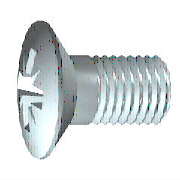
# Autodesk Inventor part: AS 1427 - M6 x 16
Saved by Autodesk Inventor 2016 (Build 200138000, 138)
## iProperties
Created: 2015-02-19
Part Number: AS 1427 - M6 x 16
Material: Steel, Mild
Description: Phillips ISO machine screws
Document SubType Name: Modeling
Standard: AS 1427
Designer: Kenneth Daniel
Standards Organization: AS
Language: en-US
Size Designation: M6 x 16
Categories: <MemberInstance><Categories><Category DisplayName="Fasteners" InternalName="e4da775c-781d-43d5-af7c-5136215cf5a6" Mnemonic="FSTN"><Category DisplayName="Bolts" InternalName="536e6df0-f778-49ac-b2f2-25c71d2aa0b2" Mnemonic="SCRW"><CategoryParameter DisplayName="Nominal Diameter Designation" InternalName="03caf894-eafd-4c09-a035-916ac084b87b" Mnemonic="nomdiadesig"/><CategoryParameter DisplayName="Nominal Length" InternalName="238ecbaf-3e6c-45dd-aa95-4068c8e0fd02" Mnemonic="nomlen"/><CategoryParameter DisplayName="Thread Designation" InternalName="586d5e89-370a-4089-914f-0110033585c7" Mnemonic="thrdesign"/><CategoryParameter DisplayName="Thread Series Designation" InternalName="87c5849c-b3a5-4c3e-9c9b-2feecef9be86" Mnemonic="thrserdsgn"/><CategoryParameter DisplayName="Nominal Diameter" InternalName="8bbe3f8e-44cf-40a9-a251-3a6edc8168d6" Mnemonic="nomdia"/><CategoryParameter DisplayName="Thread Type" InternalName="b4bbb7bc-d6aa-4c9f-a9a9-4152b9f6fe49" Mnemonic="thrtype"/><CategoryParameter DisplayName="Thread Pitch" InternalName="bb82302e-82d8-4176-8fc1-c5d7bb17d5ad" Mnemonic="pitch1"/><CategoryParameter DisplayName="Threads per Unit" InternalName="bdc6e7d2-ffd0-4d9c-a173-16b95ebb912d" Mnemonic="thrperunit1"/><CategoryParameter DisplayName="Thread Class" InternalName="ebc0d23b-2cc6-4d2a-b376-d52aae53bab6" Mnemonic="thrclss"/><Category DisplayName="Countersunk" InternalName="49656530-5684-4604-a233-68d537625f23" Mnemonic="CSSCRW"><CategoryParameter DisplayName="Type" InternalName="161b33bb-bee3-4fab-a17d-97511dff40f0" Mnemonic="type"/><CategoryParameter DisplayName="Thread Length" InternalName="207f0278-6dec-43ab-bffc-1c6d03e64de4" Mnemonic="thrlen"/><CategoryParameter DisplayName="Grip Length" InternalName="2fff3de5-ce2a-45fd-9425-99ddc9dff352" Mnemonic="grplen"/><CategoryParameter DisplayName="Property Class" InternalName="5249b721-5ecc-4781-a2e8-d7e3bda3ecca" Mnemonic="propclss"/><CategoryParameter DisplayName="Head Height" InternalName="57526df9-da71-45fb-acb4-1d0529a34778" Mnemonic="headh"/><CategoryParameter DisplayName="Shank Diameter" InternalName="7ece923f-d8ee-40d5-83f8-980cad520964" Mnemonic="grpdia"/><CategoryParameter DisplayName="Head Diameter" InternalName="a509cd31-06d1-44c5-b54e-d7a695352906" Mnemonic="headdia"/><CategoryParameter DisplayName="Head Angle" InternalName="dbcfc1e0-7990-403e-bc2e-90d1c639222a" Mnemonic="headang"/></Category></Category></Category><Category DisplayName="DataType" InternalName="23b78d0f-2648-40c6-8793-ca6db495c9e8" Mnemonic="DATATYPE"><CategoryParameter DisplayName="DisplayName" InternalName="05415f3d-3907-474b-a020-eb9d644f4cf3" Mnemonic="DISPLAYNAME"/><CategoryParameter DisplayName="Standard" InternalName="0c0a119c-1e12-4c84-803f-101930972f5e" Mnemonic="STANDARD"/><CategoryParameter DisplayName="Description" InternalName="13903e3d-64b1-4950-80da-f627842ea37f" Mnemonic="DESCRIPTION"/><CategoryParameter DisplayName="Designation" InternalName="2675968c-4ce5-49e0-a4f5-552d29089031" Mnemonic="DESIGNATION"/><CategoryParameter DisplayName="Default Row" InternalName="2af9ec52-faaa-4026-b378-f9fa4afca842" Mnemonic="DEFAULTROW"/><CategoryParameter DisplayName="Folder Name" InternalName="3f06958e-8713-4116-9be7-ed6184ecc97b" Mnemonic="FOLDERNAME"/><CategoryParameter DisplayName="Revision Guid" InternalName="45a75005-10b1-4dfc-8d6d-dfe629f0b93c" Mnemonic="REVISIONGUID"/><CategoryParameter DisplayName="FileName" InternalName="8b46a4cc-9585-4fed-90c3-899f57e09a73" Mnemonic="FILENAME"/><CategoryParameter DisplayName="StdsOrg" InternalName="8f5914e1-4693-403f-8ab5-d37768198c9d" Mnemonic="STDSORG"/><CategoryParameter DisplayName="Family Version" InternalName="914462f6-6e19-4b14-ba84-155b9680b1d0" Mnemonic="FAMILYREVISION"/><CategoryParameter DisplayName="Standard Revision" InternalName="91d5a463-65c2-4fde-b823-3b7fea5e8e17" Mnemonic="STANDARDREVISION"/><CategoryParameter DisplayName="Member Revision" InternalName="a65d44b9-392f-4f4f-857b-e4b3d54996fe" Mnemonic="MEMBERREVISION"/><CategoryParameter DisplayName="ClipFormat" InternalName="bc51e27b-3422-4e78-93ef-cec197ddf230" Mnemonic="CLIPFORMAT"/><CategoryParameter DisplayName="Manufacturer" InternalName="cd6c7a72-a28a-4e50-99a9-2c7f4e13e5ad" Mnemonic="MANUFACTURER"/><CategoryParameter DisplayName="InternalName" InternalName="cf1d0246-76d9-4b4a-8305-fa0409afb5c1" Mnemonic="INTERNALNAME"/><CategoryParameter DisplayName="IsMetric" InternalName="e2385c5b-1ea4-4823-96a8-8de651266ec3" Mnemonic="ISMETRIC"/><Category DisplayName="Part" InternalName="c0e0b642-3bcb-4cc8-9e80-f96d35c4afa4" Mnemonic="PART"><CategoryParameter DisplayName="Part Number" InternalName="016b6077-bfbe-49bd-92c9-d8d59c39c941" Mnemonic="PARTNUMBER"/><CategoryParameter DisplayName="Stock Number" InternalName="4dba7c1c-e26c-444e-836c-b08b433409a8" Mnemonic="STOCKNUMBER"/><CategoryParameter DisplayName="Material Key" InternalName="5c9a8adb-dd2b-4535-b97f-0a94a95fe41f" Mnemonic="MATERIALKEY"/><CategoryParameter DisplayName="Material" InternalName="818a152a-d3c3-49ca-80ee-df7d91421b8e" Mnemonic="MATERIAL"/></Category></Category><Category DisplayName="LegacyMap" InternalName="cd87c42b-3e48-431e-b5c0-1cbeb14dfe77" Mnemonic="LEGACYMAP"><CategoryParameter DisplayName="unique DA member ID" InternalName="0918ad47-427f-4fed-ae26-24c81c58f590" Mnemonic="DACOOKIE"/><CategoryParameter DisplayName="Merge11 ID" InternalName="0ee8fb18-e2ed-4f39-96f6-1f4b5f50aa71" Mnemonic="MERGE11"/><CategoryParameter DisplayName="unique CC member ID" InternalName="5193edd4-b2b0-4ab4-9d54-de900eee34e0" Mnemonic="CCCOOKIE"/><CategoryParameter DisplayName="Split ID" InternalName="72b5c83c-be7f-45c4-ae51-9160ea6deb26" Mnemonic="SPLIT"/><CategoryParameter DisplayName="MemberID" InternalName="8e5e0294-fc51-4c8f-b3d7-003dc5ed94f6" Mnemonic="MEMBERID"/><CategoryParameter DisplayName="CatalogName" InternalName="d99d1e27-aa94-4de2-af4c-c348882a6f4f" Mnemonic="CATALOGNAME"/><CategoryParameter DisplayName="FamilyNumber" InternalName="e705e1f4-09cb-413e-91f9-551b4188271e" Mnemonic="FAMILYNUMBER"/></Category></Categories><FamilyTemplate Id="si0144"><FamilyTemplateParameters><FamilyTemplateParameter ObjectType="kUserParameterObject" ValueType="xs:double" Id="1" ObjectReferenceKey="GUL"/><FamilyTemplateParameter ObjectType="kUserParameterObject" ValueType="xs:double" Id="2" ObjectReferenceKey="SPD"/><FamilyTemplateParameter ObjectType="kUserParameterObject" ValueType="xs:double" Id="3" ObjectReferenceKey="NLG"/><FamilyTemplateParameter ObjectType="kUserParameterObject" ValueType="xs:double" Id="4" ObjectReferenceKey="KOD"/><FamilyTemplateParameter ObjectType="kUserParameterObject" ValueType="xs:double" Id="5" ObjectReferenceKey="SBR"/><FamilyTemplateParameter ObjectType="kUserParameterObject" ValueType="xs:double" Id="6" ObjectReferenceKey="KR"/><FamilyTemplateParameter ObjectType="kUserParameterObject" ValueType="xs:double" Id="7" ObjectReferenceKey="GEL"/><FamilyTemplateParameter ObjectType="kUserParameterObject" ValueType="xs:double" Id="8" ObjectReferenceKey="KAH"/><FamilyTemplateParameter ObjectType="kUserParameterObject" ValueType="xs:double" Id="9" ObjectReferenceKey="EPV"/><FamilyTemplateParameter ObjectType="kUserParameterObject" ValueType="xs:double" Id="10" ObjectReferenceKey="THREADDIA"/><FamilyTemplateParameter ObjectType="kUserParameterObject" ValueType="xs:double" Id="11" ObjectReferenceKey="INTI"/><FamilyTemplateParameter ObjectType="kUserParameterObject" ValueType="xs:double" Id="12" ObjectReferenceKey="BDM"/><FamilyTemplateParameter ObjectType="kUserParameterObject" ValueType="xs:double" Id="13" ObjectReferenceKey="RR"/><FamilyTemplateParameter ObjectType="kUserParameterObject" ValueType="xs:double" Id="14" ObjectReferenceKey="KOH"/><FamilyTemplateParameter ObjectType="kUserParameterObject" ValueType="xs:double" Id="15" ObjectReferenceKey="TPU"/><FamilyTemplateParameter ObjectType="kUserParameterObject" ValueType="xs:double" Id="16" ObjectReferenceKey="PTC"/><FamilyTemplateParameter ObjectType="kUserParameterObject" ValueType="xs:double" Id="17" ObjectReferenceKey="SDM"/><FamilyTemplateParameter ObjectType="kUserParameterObject" ValueType="xs:double" Id="18" ObjectReferenceKey="NND"/><FamilyTemplateParameter ObjectType="kUserParameterObject" ValueType="xs:double" Id="19" ObjectReferenceKey="GD"/><FamilyTemplateParameter ObjectType="kUserParameterObject" ValueType="xs:double" Id="20" ObjectReferenceKey="SEWI"/><FamilyTemplateParameter ObjectType="kUserParameterObject" ValueType="xs:double" Id="21" ObjectReferenceKey="GAL"/><FamilyTemplateParameter ObjectType="kUserParameterObject" ValueType="xs:double" Id="22" ObjectReferenceKey="TOA"/><FamilyTemplateParameter ObjectType="kUserParameterObject" ValueType="xs:double" Id="23" ObjectReferenceKey="GD1"/><FamilyTemplateParameter ObjectType="kPropertyObject" ValueType="xs:string" Id="100" ObjectReferenceKey="{32853F0F-3444-11d1-9E93-0060B03C1CA6}" SubObjectId="52"/><FamilyTemplateParameter ObjectType="kPropertyObject" ValueType="xs:string" Id="105" ObjectReferenceKey="{32853F0F-3444-11d1-9E93-0060B03C1CA6}" SubObjectId="5"/><FamilyTemplateParameter ObjectType="kPartComponentDefinitionObject" ValueType="xs:string" Id="110" SubObjectId="Material"/><FamilyTemplateParameter ObjectType="kThreadFeatureObject" ValueType="xs:structure" Id="300" ObjectReferenceKey="1002000010000000aa0f0000000000008000000000000000" SubObjectId="ThreadInfo"><FamilyTemplateParameter ObjectType="" ValueType="xs:string" Id="301" SubObjectId="ThreadDesignation"/><FamilyTemplateParameter ObjectType="" ValueType="xs:string" Id="302" SubObjectId="ThreadClass"/><FamilyTemplateParameter ObjectType="" ValueType="xs:string" Id="303" SubObjectId="ThreadType"/></FamilyTemplateParameter></FamilyTemplateParameters></FamilyTemplate><CategoryParameterMap><ParamToTemplateMap><ParamToTemplate CategoryParameter="//CategoryParameter[@InternalName='05415f3d-3907-474b-a020-eb9d644f4cf3']" ConstantValue="AS 1427 Z Raised - Metric"/><ParamToTemplate CategoryParameter="//CategoryParameter[@InternalName='cf1d0246-76d9-4b4a-8305-fa0409afb5c1']" ConstantValue="7a313fe9-762a-49a8-869c-5b3f662deb07"/><ParamToTemplate CategoryParameter="//CategoryParameter[@InternalName='3f06958e-8713-4116-9be7-ed6184ecc97b']" ConstantValue="AS 1427(09)"/><ParamToTemplate CategoryParameter="//CategoryParameter[@InternalName='914462f6-6e19-4b14-ba84-155b9680b1d0']" ConstantValue="10"/><ParamToTemplate CategoryParameter="//CategoryParameter[@InternalName='bc51e27b-3422-4e78-93ef-cec197ddf230']" ConstantValue="CF_INVENTOR.STDPARTS"/><ParamToTemplate CategoryParameter="//CategoryParameter[@InternalName='e2385c5b-1ea4-4823-96a8-8de651266ec3']" ConstantValue="true"/><ParamToTemplate CategoryParameter="//CategoryParameter[@InternalName='13903e3d-64b1-4950-80da-f627842ea37f']" ConstantValue="Phillips ISO machine screws"/><ParamToTemplate CategoryParameter="//CategoryParameter[@InternalName='8f5914e1-4693-403f-8ab5-d37768198c9d']" ConstantValue="AS"/><ParamToTemplate CategoryParameter="//CategoryParameter[@InternalName='0c0a119c-1e12-4c84-803f-101930972f5e']" ConstantValue="AS 1427"/><ParamToTemplate CategoryParameter="//CategoryParameter[@InternalName='cd6c7a72-a28a-4e50-99a9-2c7f4e13e5ad']" TemplateParameter="104"/><ParamToTemplate CategoryParameter="//CategoryParameter[@InternalName='91d5a463-65c2-4fde-b823-3b7fea5e8e17']" TemplateParameter="103"/><ParamToTemplate CategoryParameter="//CategoryParameter[@InternalName='45a75005-10b1-4dfc-8d6d-dfe629f0b93c']" ConstantValue="7b6de92c-0d20-41fa-a3ec-45c00d3470af"/><ParamToTemplate CategoryParameter="//CategoryParameter[@InternalName='2af9ec52-faaa-4026-b378-f9fa4afca842']" ConstantValue="10"/><ParamToTemplate CategoryParameter="//CategoryParameter[@InternalName='d99d1e27-aa94-4de2-af4c-c348882a6f4f']" ConstantValue="AS"/><ParamToTemplate CategoryParameter="//CategoryParameter[@InternalName='e705e1f4-09cb-413e-91f9-551b4188271e']" ConstantValue="5"/><ParamToTemplate CategoryParameter="//CategoryParameter[@InternalName='8b46a4cc-9585-4fed-90c3-899f57e09a73']" ConstantValue="AS 1427 - M6 x 16(6) III"/><ParamToTemplate CategoryParameter="//CategoryParameter[@InternalName='a65d44b9-392f-4f4f-857b-e4b3d54996fe']" ConstantValue="0396b791-e6fc-4a64-8daf-6bfef21e989a"/><ParamToTemplate CategoryParameter="//CategoryParameter[@InternalName='2fff3de5-ce2a-45fd-9425-99ddc9dff352']" ConstantValue="5"/><ParamToTemplate CategoryParameter="//CategoryParameter[@InternalName='ebc0d23b-2cc6-4d2a-b376-d52aae53bab6']" ConstantValue="6g"/><ParamToTemplate CategoryParameter="//CategoryParameter[@InternalName='03caf894-eafd-4c09-a035-916ac084b87b']" ConstantValue="M6"/><ParamToTemplate CategoryParameter="//CategoryParameter[@InternalName='b4bbb7bc-d6aa-4c9f-a9a9-4152b9f6fe49']" ConstantValue="ISO Metric profile"/><ParamToTemplate CategoryParameter="//CategoryParameter[@InternalName='8e5e0294-fc51-4c8f-b3d7-003dc5ed94f6']" ConstantValue="220"/><ParamToTemplate CategoryParameter="//CategoryParameter[@InternalName='7ece923f-d8ee-40d5-83f8-980cad520964']" TemplateParameter="12"/><ParamToTemplate CategoryParameter="//CategoryParameter[@InternalName='2675968c-4ce5-49e0-a4f5-552d29089031']" TemplateParameter="100"/><ParamToTemplate CategoryParameter="//CategoryParameter[@InternalName='207f0278-6dec-43ab-bffc-1c6d03e64de4']" TemplateParameter="7"/><ParamToTemplate CategoryParameter="//CategoryParameter[@InternalName='a509cd31-06d1-44c5-b54e-d7a695352906']" TemplateParameter="4"/><ParamToTemplate CategoryParameter="//CategoryParameter[@InternalName='57526df9-da71-45fb-acb4-1d0529a34778']" TemplateParameter="14"/><ParamToTemplate CategoryParameter="//CategoryParameter[@InternalName='818a152a-d3c3-49ca-80ee-df7d91421b8e']" TemplateParameter="110"/><ParamToTemplate CategoryParameter="//CategoryParameter[@InternalName='238ecbaf-3e6c-45dd-aa95-4068c8e0fd02']" TemplateParameter="3"/><ParamToTemplate CategoryParameter="//CategoryParameter[@InternalName='8bbe3f8e-44cf-40a9-a251-3a6edc8168d6']" TemplateParameter="18"/><ParamToTemplate CategoryParameter="//CategoryParameter[@InternalName='016b6077-bfbe-49bd-92c9-d8d59c39c941']" TemplateParameter="105"/><ParamToTemplate CategoryParameter="//CategoryParameter[@InternalName='bb82302e-82d8-4176-8fc1-c5d7bb17d5ad']" TemplateParameter="16"/><ParamToTemplate CategoryParameter="//CategoryParameter[@InternalName='dbcfc1e0-7990-403e-bc2e-90d1c639222a']" TemplateParameter="20"/><ParamToTemplate CategoryParameter="//CategoryParameter[@InternalName='586d5e89-370a-4089-914f-0110033585c7']" TemplateParameter="301"/><ParamToTemplate CategoryParameter="//CategoryParameter[@InternalName='bdc6e7d2-ffd0-4d9c-a173-16b95ebb912d']" TemplateParameter="15"/></ParamToTemplateMap></CategoryParameterMap></MemberInstance>
Density: 7.85 g/cm^3
Appearance: Semi-Polished
IsCustomPart: 0
Author: Kenneth Daniel
Autodesk Inventor part; units mm, degrees
ref_plane "YZ Plane" through (0, 0, 0) normal (1, 0, 0) x (0, 1, 0)
sketch "Sketch1" plane through (0, 0, 0) normal (0, 0, 1) x (1, 0, 0)
  line L0 (16, 0) -> (16, 3)
  line L1 (16, 3) -> (5, 3)
  line L2 (3.9624, 5.08) -> (3.9624, 5.08)
  line L3 (3, 2.3865) -> (0.1365, 5.25)
  line L4 (0.1365, 5.25) -> (0, 5.25)
  arc A0 (0, 5.25) -> (-1.5, 0) centre (8.4375, 0) ccw
  line L5 (-1.5, 0) -> (-1.5, 5.25)
  line L6 (-0.9364, 3.299) -> (0.4274, 2.619)
  line L7 (0.4274, 2.619) -> (1.82, 0)
  line L8 (1.82, 0) -> (16, 0)
  line L9 (-5.4412, 0) -> (19.5735, 0) projected
  line L10 (0, -1.071) -> (0, 6.426) projected
  line L11 (0, 5.25) -> (0, 0) construction
  line L12 (-0.9364, 3.299) -> (-1.5, 3.58) construction
  line L13 (0, 5.25) -> (-1.5, 5.25)
  line L14 (3, 2.3865) -> (4.3866, 2.3865)
  line L15 (4.3866, 2.3865) -> (5, 3)
  line L16 (5, 3) -> (2.3865, 3) construction
  dimension "d0" = 16
  dimension "d2" = 1.5
  dimension "d3" = 6
  dimension "d4" = 3.32
  dimension "d22" = 7.16
  dimension "d23" = 10.5
  dimension "d25" = 45
  dimension "d26" = 62
  dimension "d27" = 26.5
  dimension "d31" = 4.7731
  dimension "d32" = 11
  dimension "d33" = 0.6135
  dimension "d34" = 3
  constraints: 30 end point, 5 parallel, 4 collinear, 4 point on circle, 4 point on line, 3 perpendicular, 1 centre point, 1 horizontal, 1 tangent
  measures "d0" distance from line of L0 L4.end
  measures "d2" horizontal distance of L5.start L4.end
  measures "d3" diameter of L1 L8
  measures "d4" distance from line of L7.end L5
  measures "d22" diameter of L12.end L8
  measures "d23" diameter of L4 L8
  measures "d25" angle of L3 L8
  measures "d26" angle of L7 L8
  measures "d27" angle of L6 L8
  measures "d31" diameter of L14 L8
  measures "d32" distance of L0.end L1.end
  measures "d33" horizontal distance of L14.end L1.end
  measures "d34" distance from line of L3.start L11
revolve "Body" add sketch "Sketch1" angle 360 about axis through (1.82, 0, 0) along (1, 0, 0) contours L8 L7 L6 L10 L4 L3 L14 L15 L1 L0 | L6 A0 L10
ref_plane "Work Plane1" through (-1.5, 0, 0) normal (1, 0, 0) x (0, 1, 0)
sketch "Sketch2" plane through (-1.5, 0, 0) normal (1, 0, 0) x (0, 1, 0)
  circle A0 centre (0, 0) radius 5.25 projected
  line L0 (-7.6391, 0) -> (9.0848, 0) projected
  line L1 (0, -7.6391) -> (0, 9.0848) projected
  line L2 (0, 3.58) -> (0, 0) construction
  line L3 (0, 0) -> (3.58, 0) construction
  arc A1 (1.432, 0) -> (0, 1.432) centre (0, 0) ccw construction
  line L4 (0, 0) -> (6.6957, 6.6957) construction
  line L5 (0.395, 3.5581) -> (0.3974, 1.7453)
  line L6 (3.5581, 0.395) -> (1.7453, 0.3974)
  arc A2 (0.3974, 1.7453) -> (1.351, 1.351) centre (0.956, 1.7461) ccw
  arc A3 (1.351, 1.351) -> (1.7453, 0.3974) centre (1.7461, 0.956) ccw
  arc A4 (3.58, 0) -> (3.5581, 0.395) centre (0, 0) ccw
  arc A5 (0.395, 3.5581) -> (0, 3.58) centre (0, 0) ccw
  arc A6 (3.5581, 0.395) -> (0.395, 3.5581) centre (0, 0) ccw
  line L7 (0.395, -3.5581) -> (0.3974, -1.7453)
  line L8 (3.5581, -0.395) -> (1.7453, -0.3974)
  arc A7 (1.351, -1.351) -> (0.3974, -1.7453) centre (0.956, -1.7461) ccw
  arc A8 (1.7453, -0.3974) -> (1.351, -1.351) centre (1.7461, -0.956) ccw
  arc A9 (3.5581, -0.395) -> (3.58, 0) centre (0, 0) ccw
  arc A10 (0, -3.58) -> (0.395, -3.5581) centre (0, 0) ccw
  arc A11 (0.395, -3.5581) -> (3.5581, -0.395) centre (0, 0) ccw
  line L9 (-0.395, 3.5581) -> (-0.3974, 1.7453)
  line L10 (-3.5581, 0.395) -> (-1.7453, 0.3974)
  arc A12 (-1.351, 1.351) -> (-0.3974, 1.7453) centre (-0.956, 1.7461) ccw
  arc A13 (-1.7453, 0.3974) -> (-1.351, 1.351) centre (-1.7461, 0.956) ccw
  arc A14 (-3.5581, 0.395) -> (-3.58, 0) centre (0, 0) ccw
  arc A15 (0, 3.58) -> (-0.395, 3.5581) centre (0, 0) ccw
  arc A16 (-0.395, 3.5581) -> (-3.5581, 0.395) centre (0, 0) ccw
  arc A17 (-0.395, -3.5581) -> (0, -3.58) centre (0, 0) ccw
  arc A18 (-3.5581, -0.395) -> (-0.395, -3.5581) centre (0, 0) ccw
  arc A19 (-3.58, 0) -> (-3.5581, -0.395) centre (0, 0) ccw
  line L11 (-3.5581, -0.395) -> (-1.7453, -0.3974)
  line L12 (-0.395, -3.5581) -> (-0.3974, -1.7453)
  arc A20 (-0.3974, -1.7453) -> (-1.351, -1.351) centre (-0.956, -1.7461) ccw
  arc A21 (-1.351, -1.351) -> (-1.7453, -0.3974) centre (-1.7461, -0.956) ccw
  arc A22 (1.79, 0) -> (0, 1.79) centre (0, 0) ccw construction
  dimension "d6" = 45
  dimension "d7" = 2.864
  dimension "d8" = 7.16
  dimension "d9" = 0.395
  dimension "d28" = 3.58
  constraints: 46 point on circle, 25 symmetric about line, 22 centre point, 22 end point, 6 tangent, 4 coincident, 3 collinear, 3 point on line, 1 midpoint, 1 perpendicular, 22 other
  measures "d6" angle of L4 L3
  measures "d7" diameter of A1
  measures "d8" diameter of A6
  measures "d9" distance from line of L5.start L2
  measures "d28" diameter of A22
extrude "Slot" add sketch "Sketch2" along normal up to next draft 5 contours L6 A3 A2 L5 A6 | A11 L7 A7 A8 L8 | L9 A12 A13 L10 A16 | A18 L11 A21 A20 L12
revolve "Cut" cut sketch "Sketch1" angle 360 about axis through (-10, 0, 0) along (1, 0, 0) contours L5 L13 A0
sketch "Sketch4" plane through (-1.5, 0, 0) normal (1, 0, 0) x (0, 1, 0)
  line L0 (-9.0641, 0) -> (9.0641, 0) projected
  line L1 (0, -9.0641) -> (0, 9.0641) projected
  line L2 (0, 0) -> (6.4744, 6.4744) construction
  circle A0 centre (0, 0) radius 0.1975 construction
  line L3 (0, 0) -> (6.4744, -6.4744) construction
  line L4 (0, 0) -> (-6.4744, 6.4744) construction
  line L5 (0, 0) -> (-6.4744, -6.4744) construction
  line L6 (2.5314, 2.5314) -> (0, 0.1975)
  line L7 (-2.5314, -2.5314) -> (0, -0.1975)
  line L8 (2.5314, 2.5314) -> (0.1975, 0)
  line L9 (2.5314, -2.5314) -> (0, -0.1975)
  circle A1 centre (0, 0) radius 3.58 construction
  line L10 (-2.5314, -2.5314) -> (-0.1975, 0)
  line L11 (2.5314, -2.5314) -> (0.1975, 0)
  line L12 (0, 0.1975) -> (-2.5314, 2.5314)
  line L13 (-2.5314, 2.5314) -> (-0.1975, 0)
  dimension "d16" = 0.395
  dimension "d20" = 45
  dimension "d64" = 2.5314
  constraints: 26 end point, 7 point on circle, 7 point on line, 3 symmetric about line, 2 centre point, 2 coincident, 2 perpendicular, 3 other
  measures "d16" diameter of A0
  measures "d20" angle of L2 L0
  measures "d64" distance from line of L0 L6.start
extrude "Star Cut" cut sketch "Sketch4" along normal blind 3 draft -10
fillet "Fillet1" radius 0.158 5 edges at (-0.9364, 3.2945, -0.1733) (-0.9364, 3.2945, 0.1733) (-0.9364, 0, 3.299) (-0.9364, -3.299, 0) (-0.9364, 0, -3.299)
thread "Thread" size "M6x1" class "6g" standard "ISO Metric profile" length 11
chamfer "Chamfer1" distance 0.6135 distance2 0.6136 1 edges at (16, -3, 0) measured on face at (16, -0.5525, -1.8157)
ref_plane "Work Plane3" through (3.0462, 0, 0) normal (0, 1, 0) x (1, 0, 0)
equation "\"d7\" = 0.4 * SDM"
equation "\"d8\" = SDM"
equation "\"d9\" = 0.5 * SBR"
equation "\"d28\" = 0.5 * SDM"
equation "\"d16\" = 0.5 * SBR"
equation "\"d64\" = 0.353553 * SDM"
equation "\"d17\" = KOH"
equation "\"d0\" = NLG"
equation "\"d2\" = KAH"
equation "\"d3\" = GD"
equation "\"d4\" = INTI"
equation "\"d22\" = SDM"
equation "\"d23\" = KOD"
equation "\"d25\" = 0.5 * SEWI"
equation "\"d31\" = BDM"
equation "\"d32\" = GEL"
equation "\"d33\" = GAL"
equation "\"d34\" = KOH"
equation "\"d30\" = 0.2 * SBR"
equation "\"d10\" = GEL"
equation "\"d12\" = -0.5 * SPD + 0.5 * GD"
equation "\"GD\" = NND"
equation "\"NLG\" = 16"
equation "\"GEL\" = 11"
equation "\"KOD\" = 10.5"
equation "\"KOH\" = 3"
equation "\"SDM\" = 7.16"
equation "\"INTI\" = 3.32"
equation "\"SBR\" = 0.79"
equation "\"GAL\" = 0.61345 * PTC"
equation "\"GUL\" = 0.61345 * PTC"
equation "\"KAH\" = 1.5"
equation "\"SPD\" = NND - 1.2269 * PTC"
equation "\"BDM\" = NND - 1.2269 * PTC"
equation "\"SEWI\" = 90deg"
equation "\"d5\" = -KAH"
equation "\"KR\" = 13.5"
equation "\"EPV\" = 6"
equation "\"THREADDIA\" = 6"
equation "\"RR\" = 12"
equation "\"PTC\" = 1"
equation "\"NND\" = 6"
equation "\"TOA\" = 30deg"
equation "\"GD1\" = THREADDIA - 1.2269 * PTC"
body "Solid1"
